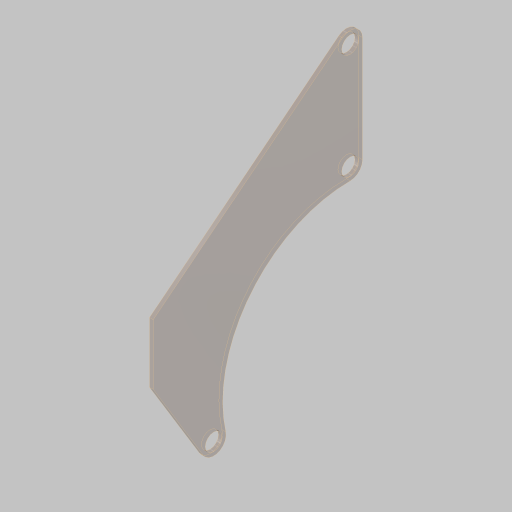
# Autodesk Inventor part: GP4-001
Saved by Autodesk Inventor 2023.5 (Build 275446000, 446)
## iProperties
Created: 2025-01-28
Part Number: GP4-001
Material: Polycarbonate, Smoke
Document SubType Name: Modeling
Designer: slick
Density: 1.2 g/cm^3
Appearance: Polycarbonate - Smoked
Author: slick
Autodesk Inventor part; units mm, degrees
ref_plane "YZ Plane" through (0, 0, 0) normal (1, 0, 0) x (0, 1, 0)
ref_plane "XZ Plane" through (0, 0, 0) normal (0, 1, 0) x (-1, 0, 0)
ref_plane "XY Plane" through (0, 0, 0) normal (0, 0, 1) x (1, 0, 0)
sketch "Sketch1" plane through (0, 0, 0) normal (1, 0, 0) x (0, 1, 0)
  circle A0 centre (0, 0) radius 203.2 construction
  circle A1 centre (234.95, 0) radius 38.1 construction
  circle A2 centre (234.95, 0) radius 31.75 construction
  circle A3 centre (-50.8, 229.3924) radius 38.1 construction
  circle A4 centre (-50.8, 229.3924) radius 31.75 construction
  circle A5 centre (412.75, 0) radius 38.1 construction
  circle A6 centre (412.75, 0) radius 31.75 construction
  line L0 (381, 150.8125) -> (266.7, 150.8125) construction
  line L1 (266.7, 150.8125) -> (266.7, -150.8125) construction
  line L2 (266.7, -150.8125) -> (381, -150.8125) construction
  line L3 (381, -150.8125) -> (381, 150.8125) construction
  line L4 (381, 150.8125) -> (266.7, -150.8125) construction
  line L5 (266.7, 150.8125) -> (381, -150.8125) construction
  point P0 (323.85, 0)
  dimension "d0" = 406.4
  dimension "d1" = 76.2
  dimension "d2" = 6.35
  dimension "d4" = 114.3
  dimension "d5" = 301.625
  dimension "d6" = 50.8
  constraints: 12 end point, 7 centre point, 4 equal radius, 4 tangent, 3 horizontal alignment, 2 coincident, 2 midpoint, 2 parallel, 1 horizontal, 1 perpendicular
  measures "d0" diameter of A0
  measures "d1" diameter of A1
  measures "d2" radial gap between concentric circles of A1 A2
  measures "d4" distance of L2.end L1.end
  measures "d5" distance of L1.end L0.end
  measures "d6" horizontal distance of A3.centre point (0, 0)
sketch "Sketch2" plane through (0, 0, 0) normal (1, 0, 0) x (0, 1, 0)
  circle A0 centre (0, 0) radius 203.2 construction
  circle A1 centre (234.95, 0) radius 38.1 construction
  circle A2 centre (234.95, 0) radius 31.75 construction
  circle A3 centre (-50.8, 229.3924) radius 38.1 construction
  circle A4 centre (-50.8, 229.3924) radius 31.75 construction
  circle A5 centre (412.75, 0) radius 38.1 construction
  circle A6 centre (412.75, 0) radius 31.75 construction
  line L0 (381, 150.8125) -> (266.7, 150.8125) construction
  line L1 (266.7, 150.8125) -> (266.7, -150.8125) construction
  line L2 (266.7, -150.8125) -> (381, -150.8125) construction
  line L3 (381, -150.8125) -> (381, 150.8125) construction
  line L4 (381, 150.8125) -> (266.7, -150.8125) construction
  line L5 (266.7, 150.8125) -> (381, -150.8125) construction
  circle A7 centre (412.75, 0) radius 14.2875
  circle A8 centre (234.95, 0) radius 14.2875
  circle A9 centre (-50.8, 229.3924) radius 14.2875
  circle A10 centre (412.75, 0) radius 20.6375 construction
  circle A11 centre (234.95, 0) radius 20.6375 construction
  circle A12 centre (-50.8, 229.3924) radius 20.6375 construction
  line L6 (412.75, -20.6375) -> (234.95, -20.6375)
  arc A13 (214.3125, 0) -> (-46.3378, 209.243) centre (0, 0) ccw
  line L7 (177.8, 330.9924) -> (76.2, 330.9924)
  line L8 (177.8, 330.9924) -> (428.9497, 12.7858)
  line L9 (76.2, 330.9924) -> (-61.5431, 247.0132)
  arc A14 (412.75, -20.6375) -> (428.9497, 12.7858) centre (412.75, 0) ccw
  arc A15 (214.3125, 0) -> (234.95, -20.6375) centre (234.95, 0) ccw
  arc A16 (-61.5431, 247.0132) -> (-46.3378, 209.243) centre (-50.8, 229.3924) ccw
  point P0 (323.85, 0)
  dimension "d7" = 28.575
  dimension "d9" = 6.35
  dimension "d10" = 101.6
  dimension "d11" = 101.6
  dimension "d12" = 76.2
  constraints: 14 point on circle, 10 centre point, 9 coincident, 8 end point, 4 equal radius, 4 tangent, 2 horizontal
  measures "d7" diameter of A7
  measures "d9" radial gap between concentric circles of A7 A10
  measures "d10" distance of L7.start L7.end
  measures "d11" vertical distance of point (-50.8, 229.392) L7.end
  measures "d12" horizontal distance of point (0, 0) L7.end
extrude "Extrusion1" add sketch "Sketch2" along normal blind 6.35
body "Solid1"
